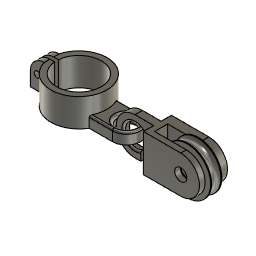
LightStandMount v4 (Autodesk Fusion 360 design; units mm, degrees)
Autodesk Fusion 360 part; units mm, degrees
note: some values were not read from the file. Set by a fixed rule: which sketch regions a step uses.
sketch "Sketch1" plane through (0, 0, 0) normal (0, 0, 1) x (1, 0, 0) in component "Mount"
  circle A0 centre (0, 0) radius 12
  circle A1 centre (0, 0) radius 15
  line L0 (0, 0) -> (-35, 0) construction
  line L1 (-11.9583, 1) -> (-14.9666, 1)
  line L2 (-11.9583, -1) -> (-14.9666, -1)
  line L3 (-14.9666, 1) -> (-21.9666, 1)
  line L4 (-21.9666, 1) -> (-21.9666, 4)
  line L5 (-21.9666, 4) -> (-14.4568, 4)
  line L6 (-21.9666, -4) -> (-14.4568, -4)
  line L7 (-21.9666, -1) -> (-21.9666, -4)
  line L8 (-14.9666, -1) -> (-21.9666, -1)
  line L9 (12.9904, 7.5) -> (32.9904, 7.5)
  line L10 (32.9904, 7.5) -> (32.9904, -7.5)
  line L11 (32.9904, -7.5) -> (12.9904, -7.5)
  dimension "d1" = 24
  dimension "d2" = 3
  dimension "d3" = 1
  dimension "d4" = 7
  dimension "d5" = 3
  dimension "d6" = 20
  dimension "d7" = 15
  dimension "d8" = 7.5
  constraint coincident A0.centre A1.centre
  constraint horizontal L0
  constraint coincident A0 L1.start
  constraint coincident A1 L1.end
  constraint parallel L0 L1
  constraint symmetric L0 L1.start L2.start
  constraint symmetric L0 L1.end L2.end
  constraint parallel L1 L3
  constraint perpendicular L3 L4
  constraint coincident A1 L5.end
  constraint perpendicular L4 L5
  constraint symmetric L0 L3.end L7.start
  constraint symmetric L0 L4.end L6.start
  constraint symmetric L0 L5.end L6.end
  constraint coincident A1 L9.start
  constraint horizontal L9
  constraint perpendicular L9 L10
  constraint coincident A1 L11.end
  constraint perpendicular L10 L11
  measures "d1" diameter of A0
  measures "d3" distance of L0 L1
  measures "d4" distance of L1.end L3.end
  measures "d5" distance of L3.end L4.end
  measures "d6" distance of L9.start L9.end
  measures "d7" distance of L9.end L10.end
  measures "d8" distance of L0 L9
extrude "Extrude1" add sketch "Sketch1" along normal blind 15 contours A0 A1 L1 L2 | A1 L3 L4 L5 | A1 L6 L7 L8 picked at (11.5885, 7.8068) makes body 1 in component "Mount"
extrude "Extrude2" add sketch "Sketch1" along normal blind 6 contours A1 L9 L10 L11 bodies 1 in component "Mount"
sketch "Sketch2" plane through (0, 0, 6) normal (0, 0, 1) x (-1, 0, 0) in component "Mount"
  line L0 (-32.9904, 7.5) -> (-32.9904, -7.5)
  line L1 (-32.9904, -7.5) -> (-12.9904, -7.5)
  arc A0 (-12.9904, 7.5) -> (-12.9904, -7.5) centre (0, 0) ccw
  line L2 (-12.9904, 7.5) -> (-32.9904, 7.5)
  line L3 (-32.9904, -7.5) -> (-17.9904, 7.5) construction
  line L4 (-32.9904, -7.5) -> (-12.6364, -7.5) construction
  line L5 (-32.9904, 7.5) -> (-17.9904, -7.5) construction
  line L6 (-32.9904, 7.5) -> (-12.6364, 7.5) construction
  circle A1 centre (-25.4904, 0) radius 5
  dimension "d13" = 45
  dimension "d14" = 45
  dimension "d15" = 10
  constraint horizontal L4
  constraint coincident L0.end L1.start
  constraint coincident L2 L3.end
  constraint horizontal L6
  constraint coincident L0.start L2.end
  constraint coincident L4 L5.end
  constraint midpoint L3 A1.centre
  measures "d13" angle of L3 L4
  measures "d14" angle of L5 L6
  measures "d15" diameter of A1
extrude "Extrude3" cut sketch "Sketch2" against normal blind 10 contours A1 bodies 1 in component "Mount"
fillet "Fillet1" radius 1.5 2 edges at (30.152, -1.8081, 6) (30.152, 1.8081, 0) on bodies 1 in component "Mount"
fillet "Fillet2" radius 7.5 2 edges at (32.9904, -7.5, 3) (32.9904, 7.5, 3) on bodies 1 in component "Mount"
fillet "Fillet3" radius 1 3 edges at (19.2404, 7.5, 6) (32.9904, 0, 6) (19.2404, -7.5, 6) on bodies 1 in component "Mount"
sketch "Sketch3" plane through (0, -4, 0) normal (0, -1, 0) x (1, 0, 0) in component "Mount"
  line L0 (-21.9666, 0) -> (-14.4568, 0)
  line L1 (-14.4568, 0) -> (-14.4568, 15)
  line L2 (-14.4568, 15) -> (-21.9666, 15)
  line L3 (-21.9666, 15) -> (-21.9666, 0)
  circle A0 centre (-18.2117, 7.5) radius 1.65
  line L4 (-21.9666, 7.5) -> (-14.4568, 7.5) construction
  dimension "d24" = 3.3
  constraint midpoint L3 L4.start
  constraint midpoint L1 L4.end
  constraint coincident A0.centre L4
  constraint midpoint A0.centre L4
  measures "d24" diameter of A0
extrude "Extrude4" cut sketch "Sketch3" against normal blind 8 contours A0 bodies 1 in component "Mount"
fillet "Fillet4" radius 7.5 2 edges at (-21.9666, 2.5, 15) (-21.9666, -2.5, 15) on bodies 1 in component "Mount"
copy_body "CutPasteBodies1" bodies 1 removing the originals makes body 2 in component "Mount"
sketch "Sketch1 (2)" plane through (0, 0, 0) normal (0, 1, 0) x (1, 0, 0) in component "Housing"
  line L0 (22, -13) -> (72, -13)
  line L1 (72, -13) -> (72, 7)
  line L2 (72, 7) -> (22, 7)
  line L3 (22, 7) -> (22, -13)
  line L4 (72, -13) -> (42, -13)
  line L5 (42, -13) -> (42, 7)
  line L6 (42, 7) -> (72, 7)
  line L7 (72, 7) -> (72, -13)
  dimension "d29" = 22
  dimension "d30" = 20
  dimension "d31" = 7
  dimension "d32" = 50
  dimension "d33" = 30
  constraint horizontal L0
  constraint vertical L1
  constraint horizontal L2
  constraint vertical L3
  constraint horizontal L4
  constraint vertical L5
  constraint horizontal L6
  constraint vertical L7
  measures "d29" distance of origin L3
  measures "d30" distance of L0 L2
  measures "d31" distance of origin L2
  measures "d32" distance of L1 L3
  measures "d33" distance of L0.end L4.end
extrude "Extrude1'" add sketch "Sketch1 (2)" along normal mid plane 15 separate body contours L0 L1 L2 L4 L5 L6 L7 makes body 3 in component "Housing"
extrude "Extrude2'" add sketch "Sketch1 (2)" along normal mid plane 4 contours L0 L2 L3 L5 bodies 3 in component "Housing"
sketch "Sketch1 (1)" plane through (0, -2, 0) normal (0, -1, 0) x (1, 0, 0) in component "Housing"
  line L0 (42, -7) -> (42, 13)
  line L1 (42, 13) -> (22, 13)
  line L2 (22, 13) -> (22, -7)
  line L3 (22, -7) -> (42, -7)
  circle A0 centre (32, 3) radius 6
  dimension "d40" = 12
  dimension "d41" = 10
  dimension "d42" = 10
  measures "d40" diameter of A0
  measures "d41" distance of L1 A0.centre
  measures "d42" distance of L2 A0.centre
extrude "Extrude3'" cut sketch "Sketch1 (1)" against normal blind 4 contours A0 bodies 3 in component "Housing"
fillet "Fillet1'" radius 10 2 edges at (22, 0, 13) (22, 0, -7) on bodies 3 in component "Housing"
sketch "Sketch2 (2)" plane through (0, -2, 0) normal (0, -1, 0) x (1, 0, 0) in component "Housing"
  arc A0 (32, 13) -> (32, -7) centre (32, 3) ccw
  line L0 (32, -7) -> (42, -7)
  line L1 (42, -7) -> (42, 13)
  line L2 (42, 13) -> (32, 13)
  circle A1 centre (32, 3) radius 6
  line L3 (35.1525, 1.8205) -> (37.7525, 1.8205)
  line L4 (37.7525, 1.8205) -> (37.7525, -10.0619)
  line L5 (37.7525, -10.0619) -> (35.1525, -10.0619)
  line L6 (35.1525, -10.0619) -> (35.1525, 1.8205)
  dimension "d47" = 2.6
  constraint horizontal L3
  constraint vertical L4
  constraint horizontal L5
  constraint vertical L6
  measures "d47" distance of L3.start L3.end
extrude "Extrude4'" cut sketch "Sketch2 (2)" against normal blind 4 contours L0 A1 L4 L6 bodies 3 in component "Housing"
fillet "Fillet2'" radius 1 2 edges at (27.2341, -2, 6.645) (27.2341, 2, 6.645) on bodies 3 in component "Housing"
sketch "Sketch3 (2)" plane through (0, 0, 13) normal (0, 0, 1) x (-1, 0, 0) in component "Housing"
  line L0 (-32, -2) -> (-32, 2)
  line L1 (-32, 2) -> (-42, 2)
  line L2 (-42, 2) -> (-42, 7.5)
  line L3 (-42, 7.5) -> (-72, 7.5)
  line L4 (-72, 7.5) -> (-72, -7.5)
  line L5 (-72, -7.5) -> (-42, -7.5)
  line L6 (-42, -7.5) -> (-42, -2)
  line L7 (-42, -2) -> (-32, -2)
  line L8 (-72, -2.5) -> (-45, -2.5)
  line L9 (-45, -2.5) -> (-45, 4.5)
  line L10 (-45, 4.5) -> (-72, 4.5)
  line L11 (-72, 4.5) -> (-72, -2.5)
  dimension "d52" = 5
  dimension "d53" = 3
  dimension "d54" = 3
  constraint horizontal L8
  constraint vertical L9
  constraint horizontal L10
  constraint vertical L11
  constraint coincident L4 L8.start
  measures "d52" distance of L5 L8
  measures "d53" distance of L3 L10
  measures "d54" distance of L6 L9
extrude "Extrude5" cut sketch "Sketch3 (2)" against normal blind 20 contours L4 L8 L9 L10 L11 bodies 3 in component "Housing"
fillet "Fillet3'" radius 10 4 edges at (72, -6, 13) (72, 5, 13) (72, 5, -7) (72, -6, -7) on bodies 3 in component "Housing"
sketch "Sketch4" plane through (0, -7.5, 0) normal (0, -1, 0) x (1, 0, 0) in component "Housing"
  arc A0 (62, -7) -> (62, 13) centre (62, 3) ccw
  line L0 (62, 13) -> (42, 13)
  line L1 (42, 13) -> (42, -7)
  line L2 (42, -7) -> (62, -7)
  circle A1 centre (62, 3) radius 3.25
  dimension "d59" = 6.5
  constraint concentric A0 A1
  measures "d59" diameter of A1
extrude "Extrude6" cut sketch "Sketch4" against normal blind 3 contours A1 bodies 3 in component "Housing"
sketch "Sketch5" plane through (0, 7.5, 0) normal (0, 1, 0) x (-1, 0, 0) in component "Housing"
  arc A0 (-62, 13) -> (-62, -7) centre (-62, 3) ccw
  line L0 (-62, -7) -> (-42, -7)
  line L1 (-42, -7) -> (-42, 13)
  line L2 (-42, 13) -> (-62, 13)
  circle A1 centre (-62, 3) radius 3.25
  circle A2 centre (-62, 3) radius 5.8
  line L3 (-56.2, 3) -> (-59.1, 8.0229)
  line L4 (-59.1, 8.0229) -> (-64.9, 8.0229)
  line L5 (-64.9, 8.0229) -> (-67.8, 3)
  line L6 (-67.8, 3) -> (-64.9, -2.0229)
  line L7 (-64.9, -2.0229) -> (-59.1, -2.0229)
  line L8 (-59.1, -2.0229) -> (-56.2, 3)
  point P0 (-62, 3)
  dimension "d62" = 11.6
  constraint concentric A1 A2
  constraint coincident A2 L3.start
  constraint coincident P0 A0.centre
  measures "d62" diameter of A2
extrude "Extrude7" cut sketch "Sketch5" against normal blind 3 contours A1 | L3 L4 L5 L6 L7 L8 bodies 3 in component "Housing"
extrude "Extrude8" cut sketch "Sketch5" against normal blind 5 contours A1 bodies 3 in component "Housing"
sketch "Sketch2 (3)" plane through (0, 0, 0) normal (0, 1, 0) x (1, 0, 0) in component "Reel"
  circle A0 centre (62, -3) radius 12.5
  circle A1 centre (62, -3) radius 3.25
  dimension "d67" = 25
  constraint concentric A0 A1
  measures "d67" diameter of A0
extrude "Extrude2''" add sketch "Sketch2 (3)" along normal blind 2 and the other way blind 4 separate body makes body 4 in component "Reel"
ref_plane "WorkPlane1" through (62, -4.5, 13) normal (-1, 0, 0) x (0, -1, 0) in component "Reel"
sketch "Sketch3 (3)" plane through (62, -4.5, 13) normal (-1, 0, 0) x (0, 1, 0) in component "Reel"
  line L0 (0.5, 22.5) -> (0.5, -2.5)
  line L1 (6.5, -2.5) -> (6.5, 22.5)
  line L2 (0.5, -2.5) -> (6.5, -2.5)
  line L3 (0.5, -2.5) -> (1, -2.5)
  line L4 (6.5, -2.5) -> (6, -2.5)
  arc A0 (6, -2.5) -> (1, -2.5) centre (3.5, -3.0625) ccw
  dimension "d73" = 0.5
  dimension "d74" = 0.5
  dimension "d75" = 2.5625
  dimension "d76" = 360
  constraint coincident L1 L2.end
  constraint coincident L0.end L2.start
  constraint perpendicular L1 L2
  constraint perpendicular L0 L3
  constraint perpendicular L1 L4
  measures "d73" distance of L0.end L3.end
  measures "d74" distance of L1.start L4.end
  measures "d75" radius of A0
revolve "Revolve1" cut sketch "Sketch3 (3)" angle 360 about axis through (62, -9, 3) along (0, 1, 0) bodies 4 in component "Reel"
component "Mount" placed x (1, 0, 0) y (0, 1, 0) z (0, 0, 1) at (0, 0, 0)
component "Pully" placed x (1, 0, 0) y (0, 1, 0) z (0, 0, 1) at (0, 0, 0)
component "Housing" placed x (1, 0, 0) y (0, 1, 0) z (0, 0, 1) at (0, 0, 0) in component "Pully"
component "Reel" placed x (1, 0, 0) y (0, 1, 0) z (0, 0, 1) at (0, 0, 0) in component "Pully"
equation "d68 = 2.50 mm - 0.5 mm"
equation "d70 = 4.50 mm - 0.5 mm"
